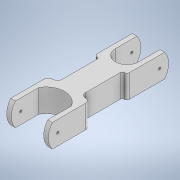
# Autodesk Inventor part: PartArmNEW
Saved by Autodesk Inventor 2022 (Build 260153000, 153)
## iProperties
Created: 2022-01-13
Part Number: PartArmNEW
Material: Generic
Document SubType Name: Modeling
Designer: nguye
Density: 1 g/cm^3
Appearance: Default
Author: nguye
Autodesk Inventor part; units mm, degrees
ref_plane "YZ Plane" through (0, 0, 0) normal (1, 0, 0) x (0, 1, 0)
ref_plane "XZ Plane" through (0, 0, 0) normal (0, 1, 0) x (-1, 0, 0)
ref_plane "XY Plane" through (0, 0, 0) normal (0, 0, 1) x (1, 0, 0)
sketch "Sketch1" plane through (0, 0, 0) normal (0, 1, 0) x (-1, 0, 0)
  line L0 (90, 0) -> (90, -90)
  line L1 (0, -90) -> (0, 0)
  line L2 (90, 0) -> (90, -90)
  line L3 (90, -90) -> (0, -90)
  line L4 (10, -180) -> (80, -180)
  line L5 (90, 0) -> (80, 0)
  line L6 (80, 0) -> (80, -90)
  line L7 (0, 0) -> (10, 0)
  line L8 (10, 0) -> (10, -90)
  line L9 (80, -270) -> (80, -180)
  line L10 (10, -270) -> (10, -180)
  line L11 (80, -270) -> (70, -270)
  line L12 (70, -270) -> (70, -180)
  line L13 (10, -270) -> (20, -270)
  line L14 (20, -270) -> (20, -180)
  line L15 (80, -90) -> (70, -90)
  line L16 (70, -180) -> (60, -180)
  line L17 (20, -180) -> (30, -180)
  line L18 (70, -180) -> (70, -90)
  line L19 (20, -180) -> (20, -90)
  line L20 (80, -270) -> (70, -270)
  line L21 (20, -270) -> (10, -270)
  line L22 (0, 0) -> (10, 0)
  line L23 (80, 0) -> (90, 0)
  line L24 (90, 0) -> (80, 0)
  line L25 (0, 0) -> (10, 0)
  line L26 (90, 0) -> (0, 0)
  line L27 (80, -270) -> (10, -270)
  dimension "d2" = 90
  dimension "d4" = 10
  dimension "d5" = 10
  constraints: 56 end point, 13 perpendicular, 8 point on line, 6 parallel, 2 collinear, 2 horizontal
  measures "d2" distance of L0.end L0.start
  measures "d4" distance of L0.start L5.end
  measures "d5" distance of L1.end L7.end
extrude "Extrusion1" add sketch "Sketch1" along normal blind 50
sketch "Sketch2" plane through (0, 50, 0) normal (0, 1, 0) x (1, 0, 0)
  arc A0 (-10, 59.3649) -> (-80, 59.3649) centre (-45, 40) ccw
  line L0 (-90, 0) -> (0, 0) projected
  line L1 (-90, 0) -> (-80, 0)
  line L2 (-80, 0) -> (-80, 59.3649)
  line L3 (0, 0) -> (-10, 0)
  line L4 (-10, 0) -> (-10, 59.3649)
  line L5 (-80, 0) -> (-10, 0)
  line L6 (-80, 270) -> (-80, 180) projected
  line L7 (-70, 270) -> (-20, 270)
  line L8 (-80, 180) -> (-80, 190)
  line L9 (-10, 180) -> (-10, 270) projected
  line L10 (-70, 270) -> (-70, 215)
  line L11 (-20, 270) -> (-20, 215)
  arc A1 (-70, 215) -> (-20, 215) centre (-45, 215) ccw
  point P0 (-90, 90)
  dimension "d18" = 10
  dimension "d19" = 10
  dimension "d25" = 10
  constraints: 18 end point, 4 point on circle, 3 point on line, 2 centre point, 1 collinear, 1 tangent
  measures "d18" distance of L0.start L1.end
  measures "d19" distance of L0.end L3.end
  measures "d25" distance of L6.end L8.end
extrude "Extrusion2" cut sketch "Sketch2" against normal blind 50
fillet "Fillet1" radius 10 1 edges at (-70, 25, -90)
fillet "Fillet2" radius 10 1 edges at (-90, 25, -90)
fillet "Fillet3" radius 10 2 edges at (-20, 25, -90) (0, 25, -90)
fillet "Fillet4" radius 5 1 edges at (-80, 25, -180)
fillet "Fillet5" radius 5 3 edges at (-70, 25, -180) (-10, 25, -180) (-20, 25, -180)
sketch "Sketch3" plane through (-90, 0, 0) normal (-1, 0, 0) x (0, 0, 1)
  line L0 (0, 0) -> (0, 50) projected
  circle A0 centre (-20, 25) radius 2.5
  arc A1 (-8.775, 0) -> (-8.775, 50) centre (-40, 25) ccw
  line L1 (-80, 0) -> (-90, 0) projected
  line L2 (-8.775, 0) -> (0, 0)
  line L3 (0, 0) -> (0, 50)
  line L4 (0, 50) -> (-8.775, 50)
  line L5 (-270, 0) -> (-270, 50) projected
  circle A2 centre (-250, 25) radius 2.5
  line L6 (-270, 50) -> (-270, 0)
  arc A3 (-261.225, 50) -> (-261.225, 0) centre (-230, 25) ccw
  line L7 (-270, 0) -> (-261.225, 0)
  line L8 (-185, 0) -> (-270, 0) projected
  line L9 (-270, 50) -> (-261.225, 50)
  line L10 (-270, 50) -> (-185, 50) projected
  point P0 (0, 25)
  point P1 (-270, 25)
  dimension "d36" = 5
  dimension "d40" = 5
  constraints: 12 end point, 4 centre point, 4 point on circle, 2 collinear, 1 horizontal, 1 parallel, 1 perpendicular
  measures "d36" diameter of A0
  measures "d40" diameter of A2
extrude "Extrusion3" cut sketch "Sketch3" against normal blind 150.25
sketch "Sketch4" plane through (-20, 0, -215) normal (-1, 0, 0) x (0, 0, 1)
  circle A0 centre (-35, 25) radius 2.5 projected
  line L0 (-45, 25) -> (-45, 32.5)
  line L1 (-45, 32.5) -> (-15, 32.5)
  line L2 (-15, 32.5) -> (-15, 17.5)
  line L3 (-15, 17.5) -> (-45, 17.5)
  line L4 (-45, 25) -> (-45, 17.5)
  point P0 (215, 0)
  dimension "d43" = 10
  dimension "d44" = 7.5
  dimension "d45" = 30
  dimension "d47" = 15
  constraints: 10 end point, 2 perpendicular, 2 vertical
  measures "d43" distance of A0.centre L0.start
  measures "d44" distance of L0.start L0.end
  measures "d45" distance of L0.end L1.end
  measures "d47" distance of L1.end L2.end
extrude "Extrusion4" cut sketch "Sketch4" against normal blind 5
sketch "Sketch5" plane through (-20, 0, -215) normal (-1, 0, 0) x (0, 0, 1)
  line L0 (-45, 17.5) -> (-45, 32.5) projected
  line L1 (-45, 32.5) -> (-45, 35)
  line L2 (-15, 17.5) -> (-45, 17.5) projected
  line L3 (-45, 17.5) -> (-45, 15)
  line L4 (-45, 15) -> (-5, 15)
  line L5 (-5, 15) -> (-5, 35)
  line L6 (-5, 35) -> (-45, 35)
  line L7 (-45, 17.5) -> (-45, 32.5)
  point P0 (215, 0)
  dimension "d50" = 2.5
  dimension "d51" = 2.5
  dimension "d52" = 40
  dimension "d53" = 20
  constraints: 12 end point, 2 vertical, 1 horizontal, 1 perpendicular
  measures "d50" distance of L0.end L1.end
  measures "d51" distance of L0.start L3.end
  measures "d52" distance of L3.end L4.end
  measures "d53" distance of L4.end L5.end
extrude "Extrusion5" cut sketch "Sketch5" against normal blind 5
body "Solid1"
